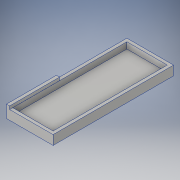
# Autodesk Inventor part: Camera Platform
Saved by Autodesk Inventor 2017 (Build 210142000, 142)
## iProperties
Created: 2016-12-06
Part Number: Camera Platform
Material: Aluminum 6061
Document SubType Name: Modeling
Designer: qupec
Density: 2.7 g/cm^3
Appearance: Aluminum - Flat
Author: qupec
Autodesk Inventor part; units mm, degrees
ref_plane "YZ Plane" through (0, 0, 0) normal (1, 0, 0) x (0, 1, 0)
ref_plane "XZ Plane" through (0, 0, 0) normal (0, 1, 0) x (-1, 0, 0)
ref_plane "XY Plane" through (0, 0, 0) normal (0, 0, 1) x (1, 0, 0)
sketch "Sketch1" plane through (0, 0, 0) normal (0, 1, 0) x (-1, 0, 0)
  line L0 (10.25, 29) -> (-10.25, 29)
  line L1 (-10.25, 29) -> (-10.25, -29)
  line L2 (-10.25, -29) -> (10.25, -29)
  line L3 (10.25, -29) -> (10.25, 29)
  line L4 (11.8375, 30.5875) -> (-11.8375, 30.5875)
  line L5 (-11.8375, 30.5875) -> (-11.8375, -30.5875)
  line L6 (-11.8375, -30.5875) -> (11.8375, -30.5875)
  line L7 (11.8375, -30.5875) -> (11.8375, 30.5875)
  point P0 (0, 0)
  dimension "d0" = 20.5
  dimension "d1" = 1.5875
  dimension "d2" = 1.5875
  dimension "d3" = 1.5875
  dimension "d4" = 1.5875
  dimension "d5" = 58
  dimension "d6" = 29
  dimension "d7" = 10.25
  constraints: 16 end point, 4 parallel, 2 horizontal, 2 perpendicular
  measures "d0" distance of L0.start L0.end
  measures "d1" distance between parallel lines of L3 L7
  measures "d2" distance between parallel lines of L1 L5
  measures "d3" distance between parallel lines of L0 L4
  measures "d4" distance between parallel lines of L6 L2
  measures "d5" distance of L2.end L0.start
  measures "d6" distance from line of point (0, 0) L0
  measures "d7" distance from line of point (0, 0) L1
extrude "Extrusion1" add sketch "Sketch1" along normal blind 3.175
sketch "Sketch2" plane through (0, 0, 0) normal (0, -1, 0) x (1, 0, 0)
  line L0 (-10.25, -29) -> (-10.25, 29) construction
  line L1 (-10.25, 29) -> (10.25, 29) construction
  line L2 (10.25, 29) -> (10.25, -29) construction
  line L3 (10.25, -29) -> (-10.25, -29) construction
  line L4 (-11.8375, 30.5875) -> (11.8375, 30.5875) projected
  line L5 (-11.8375, -30.5875) -> (-11.8375, 30.5875) projected
  line L6 (11.8375, -30.5875) -> (-11.8375, -30.5875) projected
  line L7 (11.8375, 30.5875) -> (11.8375, -30.5875) projected
  point P0 (0, 0)
extrude "Extrusion2" add sketch "Sketch2" along normal blind 1.5875
sketch "Sketch3" plane through (0, 3.175, 0) normal (0, 1, 0) x (1, 0, 0)
  line L0 (11.8375, 30.5875) -> (11.8375, -30.5875) projected
  line L1 (10.25, -29) -> (10.25, 29) projected
  line L2 (-11.8375, -30.5875) -> (-11.8375, 30.5875) projected
  line L3 (-11.8375, -30.5875) -> (-10.2373, -30.5875)
  line L4 (-10.2373, -30.5875) -> (-10.2373, -5.1875)
  line L5 (-10.2373, -5.1875) -> (-11.8375, -5.1875)
  line L6 (-11.8375, -5.1875) -> (-11.8375, -30.5875)
  point P0 (0, 0)
  dimension "d13" = 1.6002
  dimension "d14" = 25.4
  constraints: 8 end point, 2 parallel, 1 horizontal, 1 perpendicular
  measures "d13" distance of L5.end L4.end
  measures "d14" distance of L4.end L3.end
extrude "Extrusion3" add sketch "Sketch3" along normal blind 1.5875
equation "\"d2\" = d1"
equation "\"d3\" = d2"
equation "\"d4\" = d3"
equation "\"d6\" = 0.5 * d5"
equation "\"d7\" = 0.5 * d0"
body "Solid1"
